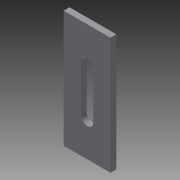
# Autodesk Inventor part: back brace mount
Saved by Autodesk Inventor 2013 (Build 170138000, 138)
## iProperties
Created: 2013-02-04
Part Number: back brace mount
Material: Generic
Document SubType Name: Sheet Metal
Designer: Arpan
Density: 1 g/cm^3
Sheet Metal Rule: Default
Author: Arpan
Autodesk Inventor part; units mm, degrees
ref_plane "YZ Plane" through (0, 0, 0) normal (1, 0, 0) x (0, 1, 0)
ref_plane "XZ Plane" through (0, 0, 0) normal (0, 1, 0) x (-1, 0, 0)
ref_plane "XY Plane" through (0, 0, 0) normal (0, 0, 1) x (1, 0, 0)
sketch "Sketch1" plane through (0, 0, 0) normal (0, 0, 1) x (1, 0, 0)
  line L0 (36.9316, 0) -> (11.5316, 0)
  line L1 (36.9316, 63.5) -> (36.9316, 0)
  line L2 (11.5316, 63.5) -> (36.9316, 63.5)
  line L3 (20.8534, 19.05) -> (20.8534, 44.45)
  arc A0 (27.6098, 44.45) -> (20.8534, 44.45) centre (24.2316, 44.45) ccw
  line L4 (27.6098, 44.45) -> (27.6098, 19.05)
  arc A1 (20.8534, 19.05) -> (27.6098, 19.05) centre (24.2316, 19.05) ccw
  line L5 (36.9316, 63.5) -> (11.5316, 63.5)
  line L6 (11.5316, 63.5) -> (11.5316, 0)
  point P0 (0, 0)
  point P1 (0, 0)
  dimension "d0" = 25.4
  measures "d0" distance of L5.end L5.start
extrude "Plate1" add sketch "Sketch1" along normal blind 3.175
equation "\"BendRadius\" = Thickness"
equation "\"BendReliefWidth\" = Thickness"
equation "\"BendReliefDepth\" = 0.5 * Thickness"
equation "\"CornerReliefSize\" = 4 * Thickness"
equation "\"MinimumRemnant\" = 2 * Thickness"
equation "\"TransitionRadius\" = BendRadius"
equation "\"JacobiRadiusSize\" = BendRadius"
equation "\"GapSize\" = Thickness"
equation "\"d1\" = BendRadius"
equation "\"Thickness\" = 3.175"
body "Solid1"
